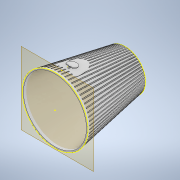
# Autodesk Inventor part: Lampshade
Saved by Autodesk Inventor 2020 (Build 240168000, 168)
## iProperties
Created: 2020-08-31
Part Number: Lampshade
Material: Generic
Document SubType Name: Modeling
Designer: samhita001
Density: 1 g/cm^3
Appearance: Default
Author: samhita001
Autodesk Inventor part; units mm, degrees
ref_plane "YZ Plane" through (0, 0, 0) normal (1, 0, 0) x (0, 1, 0)
sketch "Sketch1" plane through (0, 0, 0) normal (0, 1, 0) x (-1, 0, 0)
  line L0 (0, 0) -> (-56.25, 0)
  line L1 (0, 0) -> (0, -120)
  line L2 (0, -120) -> (-34.75, -120)
  line L3 (-34.75, -120) -> (-56.25, 0)
  line L4 (-17.375, -120) -> (-17.375, -116)
  line L5 (0, -116) -> (-25.75, -116)
  line L6 (-34.75, -120) -> (-32.45, -120)
  line L7 (-32.45, -120) -> (-25.75, -116)
  dimension "d1" = 56.25
  dimension "d2" = 120
  dimension "d3" = 34.75
  dimension "d4" = 4
  dimension "d5" = 25.75
  dimension "d6" = 2.3
  constraints: 16 end point, 2 horizontal, 2 point on line, 2 vertical, 1 midpoint, 1 parallel
  measures "d1" distance of L0.start L0.end
  measures "d2" distance of L0.start L1.end
  measures "d3" distance of L1.end L2.end
  measures "d4" distance of L4.start L4.end
  measures "d5" distance of L5.start L5.end
  measures "d6" distance of L2.end L6.end
revolve "Revolution1" add sketch "Sketch1" angle 360 about axis through (0, 0, 0) along (0, 0, -1) contours L1 L5 L7 L2 L3 L0
fillet "Fillet1" radius 8 1 edges at (-25.75, 0, -116)
fillet "Fillet2" radius 2 1 edges at (-32.45, 0, -120)
shell "Shell1" thickness 2.3 removed faces 1 at (4.1843, 21.3622, 0)
sketch "Sketch2" plane through (0, 0, 0) normal (0, 0, 1) x (1, 0, 0)
  circle A0 centre (0, 0) radius 56.25 projected
sketch "Sketch5" plane through (0, 0, -120) normal (0, 0, -1) x (-1, 0, 0)
  line L0 (-17.8318, 21.5886) -> (-18.0642, 21.6519)
  line L1 (-18.0642, 21.6519) -> (-17.9693, 21.7733)
  circle A0 centre (0, 0) radius 34.75 projected
  line L2 (-22.7, 26.2954) -> (-21.7, 26.2954) construction
  constraints: 6 end point, 1 horizontal
sketch "Sketch6" plane through (0, 0, 0) normal (0, 0, 1) x (1, 0, 0)
  circle A0 centre (0, 0) radius 56.25 projected
ref_plane "Work Plane1" through (0, 0, -4) normal (0, 0, 1) x (1, 0, 0)
sketch "Sketch14" plane through (0, 0, -120) normal (0, 0, -1) x (-1, 0, 0)
  line L0 (34.7381, 0) -> (33.7381, 0)
  line L1 (33.7381, 0.3211) -> (33.7381, -0.3211)
  line L2 (33.7381, -0.3211) -> (34.7381, -0.91)
  line L3 (34.7381, 0.91) -> (33.7381, 0.3211)
  arc A0 (34.7381, -0.91) -> (34.7381, 0.91) centre (33.4556, 0) ccw
  point P0 (0, 0)
  constraints: 8 end point, 2 point on circle, 1 centre point, 1 horizontal, 1 vertical
sketch "Sketch16" plane through (0, 0, -4) normal (0, 0, 1) x (1, 0, 0)
  line L0 (-55.5139, 0) -> (-54.5139, 0)
  line L1 (-55.2316, -0.484) -> (-55.2316, 0.547)
  line L2 (-55.2316, 0.547) -> (-56.2313, 1.4982)
  line L3 (-55.2316, -0.484) -> (-56.2313, -1.4418)
  line L4 (-56.2313, -1.4418) -> (-56.2313, 1.4982)
  point P0 (0, 0)
  dimension "d39" = 2.94
  dimension "d42" = 1.031
  constraints: 10 end point, 2 vertical, 1 horizontal
  measures "d39" distance of L3.end L2.end
  measures "d42" distance of L1.start L1.end
loft "Loft3" cut profiles "Sketch14", "Sketch16"
pattern_circular "Circular Pattern1" count 59 over 360 about axis through (0, 0, -59.5944) along (0, 0, 1) of "Loft3"
sketch "Sketch24" plane through (0, 0, 0) normal (0, 1, 0) x (-1, 0, 0)
  line L0 (-18.25, -17.0587) -> (18.25, -17.0587)
  arc A0 (10.3721, -48.9734) -> (18.25, -17.0587) centre (-40.1642, -19.5692) ccw
  arc A1 (-18.25, -17.0587) -> (-10.3721, -48.9734) centre (40.1642, -19.5692) ccw
  arc A2 (-10.3721, -48.9734) -> (10.3721, -48.9734) centre (0, -42.9384) ccw
  point P0 (0, 0)
  dimension "d74" = 36.5
  dimension "d76" = 12
  constraints: 6 point on circle, 3 centre point, 2 end point, 2 tangent, 1 horizontal
  measures "d74" distance of L0.start L0.end
  measures "d76" radius of A2
extrude "Extrusion2" add sketch "Sketch24" along normal blind 70
sketch "Sketch26" plane through (0, 0, 0) normal (1, 0, 0) x (0, 1, 0)
  line L0 (44.0702, -54.9384) -> (50.857, -17.0587)
  line L1 (34.75, -120) -> (46.4069, -54.9384) projected
  line L2 (53.1937, -17.0587) -> (53.0859, -17.0587) projected
  line L3 (46.4069, -54.9384) -> (53.1937, -17.0587)
  line L4 (0, -54.9384) -> (0, -48.9734) projected
  line L5 (44.0702, -54.9384) -> (0, -54.9384)
  line L6 (0, -48.9734) -> (0, -17.0587) projected
  line L7 (0, -54.9384) -> (0, -17.0587)
  line L8 (0, -17.0587) -> (50.857, -17.0587)
  line L9 (53.1937, -17.0587) -> (73.2872, -17.0587)
  line L10 (49.965, -17.0587) -> (70, -17.0587) projected
  line L11 (73.2872, -17.0587) -> (73.2872, -54.9384)
  line L12 (73.2872, -54.9384) -> (46.4069, -54.9384)
  line L13 (46.4069, -54.9384) -> (70, -54.9384) projected
  point P0 (0, 0)
  constraints: 16 end point, 3 collinear, 2 perpendicular, 1 horizontal, 1 parallel, 1 point on line
revolve "Revolution2" cut sketch "Sketch26" angle 360 about axis through (0, 0, -54.9384) along (0, 0, 1)
ref_plane "Work Plane9" through (1.4425, 53.1741, -17.0587) normal (0.0266931, 0.983964, -0.1763584) x (-0.9996322, 0.0271182, 0)
sketch "Sketch27" plane through (1.4425, 53.1741, -17.0587) normal (0.0266931, 0.983964, -0.1763584) x (-0.9996322, 0.0271182, 0)
  point P0 (0, 7.4101)
  point P1 (2.4288, -6.2587)
sketch "Sketch28" plane through (1.4425, 53.1741, -17.0587) normal (0.0266931, 0.983964, -0.1763584) x (-0.9996322, 0.0271182, 0)
  line L0 (-0.875, -4.9173) -> (-0.875, -16.9173)
  line L1 (1.125, -16.9173) -> (1.125, -4.9173)
  arc A0 (1.125, -4.9173) -> (-0.875, -4.9173) centre (0.125, -4.9173) ccw
  arc A1 (-0.875, -16.9173) -> (1.125, -16.9173) centre (0.125, -16.9173) ccw
  point P0 (0, 7.4101)
  dimension "d90" = 14
  dimension "d91" = 2
  constraints: 4 end point, 4 point on circle, 4 tangent, 2 centre point, 1 parallel
  measures "d91" distance between parallel lines of L0 L1
extrude "Extrusion3" add sketch "Sketch28" along normal blind 3
ref_plane "Work Plane11" through (1.5226, 56.126, -17.5877) normal (0.0266931, 0.983964, -0.1763584) x (0.9996322, -0.0271182, 0)
sketch "Sketch30" plane through (1.5226, 56.126, -17.5877) normal (0.0266931, 0.983964, -0.1763584) x (0.9996322, -0.0271182, 0)
  line L0 (0, 17.9095) -> (0, 3.9252) projected
  line L1 (-6, 5.7721) -> (6, 5.7721)
  arc A0 (6, 5.7721) -> (-6, 5.7721) centre (0, 10.9801) ccw
  point P0 (0, -7.4101)
  dimension "d88" = 12
  constraints: 2 end point, 2 point on circle, 1 centre point, 1 horizontal
  measures "d88" distance of L1.start L1.end
extrude "Extrusion4" add sketch "Sketch30" against normal blind 1
sketch "Sketch31" plane through (0, 0, -116) normal (0, 0, -1) x (-1, 0, 0)
  circle A0 centre (0, 0) radius 5
  dimension "d94" = 10
  constraints: 1 centre point, 1 coincident
  measures "d94" diameter of A0
extrude "Extrusion5" cut sketch "Sketch31" against normal through all
body "Solid1"
